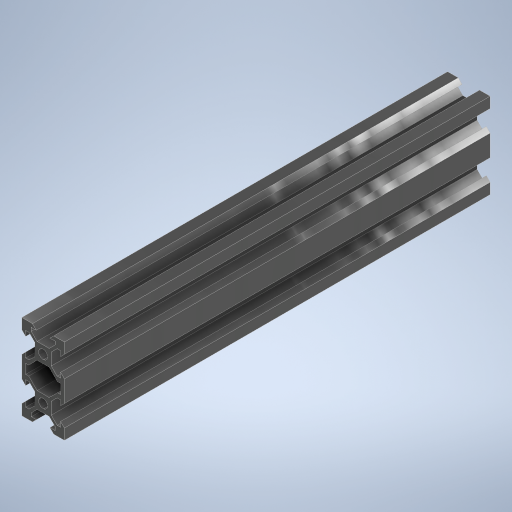
# Autodesk Inventor part: AP20x20
Saved by Autodesk Inventor 2024.2 (Build 282272000, 272)
## iProperties
Created: 2024-08-13
Part Number: AP20x20
Material: Generic
Document SubType Name: Modeling
Designer: Admin
Density: 1 g/cm^3
Appearance: Dark Gray
Author: Admin
Autodesk Inventor part; units mm, degrees
ref_plane "YZ Plane" through (0, 0, 0) normal (1, 0, 0) x (0, 1, 0)
ref_plane "XZ Plane" through (0, 0, 0) normal (0, 1, 0) x (-1, 0, 0)
ref_plane "XY Plane" through (0, 0, 0) normal (0, 0, 1) x (1, 0, 0)
sketch "Sketch1" plane through (0, 0, 0) normal (0, 0, 1) x (1, 0, 0)
  line L0 (-10, -10) -> (-5.6, -10)
  line L1 (-10, -5.6) -> (-10, -10)
  line L2 (-5.6, -10) -> (-5, -10)
  line L3 (-3.2, -8.2) -> (-5.6, -8.2)
  line L4 (-2.8351, -3.825) -> (-5.6, -6.5899)
  line L5 (-3.825, -2.8351) -> (-6.5899, -5.6)
  line L6 (0, 0) -> (0, -11) construction
  line L7 (0, 0) -> (-12, 0) construction
  line L8 (-3.2, -8.2) -> (-5, -10)
  line L9 (-6.5899, -5.6) -> (-8.2, -5.6)
  line L10 (-10, -5.6) -> (-10, -5)
  line L11 (-10, -5) -> (-8.2, -3.2)
  line L12 (-8.2, -3.2) -> (-8.2, -5.6)
  line L13 (-5.6, -8.2) -> (-5.6, -6.5899)
  arc A0 (-2.15, 0) -> (0, -2.15) centre (0, 0) ccw
  line L14 (0, 0) -> (-3.825, 0)
  line L15 (-3.825, 0) -> (-3.825, -2.8351)
  line L16 (-2.8351, -3.825) -> (0, -3.825)
  line L17 (0, -3.825) -> (0, 0)
  line L18 (-2.8351, -3.825) -> (-3.825, -3.825) construction
  line L19 (-3.825, -3.825) -> (-3.825, -2.8351) construction
  line L20 (3.825, -2.8351) -> (3.825, -3.825) construction
  line L21 (3.825, -2.8351) -> (3.825, 0)
  line L22 (3.825, -3.825) -> (2.8351, -3.825) construction
  line L23 (3.825, 0) -> (0, 0)
  line L24 (0, -3.825) -> (2.8351, -3.825)
  arc A1 (0, -2.15) -> (2.15, 0) centre (0, 0) ccw
  line L25 (0, 0) -> (0, -3.825)
  line L26 (2.8351, -3.825) -> (5.6, -6.5899)
  line L27 (0, 0) -> (0, -12) construction
  line L28 (0, 0) -> (11, 0) construction
  line L29 (3.825, -2.8351) -> (6.5899, -5.6)
  line L30 (8.2, -3.2) -> (8.2, -5.6)
  line L31 (10, -5.6) -> (10, -5)
  line L32 (8.2, -3.2) -> (10, -5)
  line L33 (8.2, -5.6) -> (6.5899, -5.6)
  line L34 (5.6, -6.5899) -> (5.6, -8.2)
  line L35 (10, -10) -> (10, -5.6)
  line L36 (5.6, -10) -> (10, -10)
  line L37 (3.2, -8.2) -> (5.6, -8.2)
  line L38 (5, -10) -> (3.2, -8.2)
  line L39 (5.6, -10) -> (5, -10)
  line L40 (2.8351, 3.825) -> (3.825, 3.825) construction
  line L41 (2.8351, 3.825) -> (0, 3.825)
  line L42 (3.825, 3.825) -> (3.825, 2.8351) construction
  line L43 (0, 3.825) -> (0, 0)
  line L44 (3.825, 0) -> (3.825, 2.8351)
  arc A2 (2.15, 0) -> (0, 2.15) centre (0, 0) ccw
  line L45 (0, 0) -> (3.825, 0)
  line L46 (3.825, 2.8351) -> (6.5899, 5.6)
  line L47 (0, 0) -> (12, 0) construction
  line L48 (0, 0) -> (0, 11) construction
  line L49 (2.8351, 3.825) -> (5.6, 6.5899)
  line L50 (3.2, 8.2) -> (5.6, 8.2)
  line L51 (5.6, 10) -> (5, 10)
  line L52 (3.2, 8.2) -> (5, 10)
  line L53 (5.6, 8.2) -> (5.6, 6.5899)
  line L54 (6.5899, 5.6) -> (8.2, 5.6)
  line L55 (10, 10) -> (5.6, 10)
  line L56 (10, 5.6) -> (10, 10)
  line L57 (8.2, 3.2) -> (8.2, 5.6)
  line L58 (10, 5) -> (8.2, 3.2)
  line L59 (10, 5.6) -> (10, 5)
  line L60 (-3.825, 2.8351) -> (-3.825, 3.825) construction
  line L61 (-3.825, 2.8351) -> (-3.825, 0)
  line L62 (-3.825, 3.825) -> (-2.8351, 3.825) construction
  line L63 (-3.825, 0) -> (0, 0)
  line L64 (0, 3.825) -> (-2.8351, 3.825)
  arc A3 (0, 2.15) -> (-2.15, 0) centre (0, 0) ccw
  line L65 (0, 0) -> (0, 3.825)
  line L66 (-2.8351, 3.825) -> (-5.6, 6.5899)
  line L67 (0, 0) -> (0, 12) construction
  line L68 (0, 0) -> (-11, 0) construction
  line L69 (-3.825, 2.8351) -> (-6.5899, 5.6)
  line L70 (-8.2, 3.2) -> (-8.2, 5.6)
  line L71 (-10, 5.6) -> (-10, 5)
  line L72 (-8.2, 3.2) -> (-10, 5)
  line L73 (-8.2, 5.6) -> (-6.5899, 5.6)
  line L74 (-5.6, 6.5899) -> (-5.6, 8.2)
  line L75 (-10, 10) -> (-10, 5.6)
  line L76 (-5.6, 10) -> (-10, 10)
  line L77 (-3.2, 8.2) -> (-5.6, 8.2)
  line L78 (-5, 10) -> (-3.2, 8.2)
  line L79 (-5.6, 10) -> (-5, 10)
  point P0 (0, 2.15)
  point P1 (2.15, 0)
  point P2 (0, -2.15)
  dimension "d16" = 10
  dimension "d19" = 3.2
  dimension "d21" = 4.4
  dimension "d22" = 4.4
  dimension "d24" = 45
  dimension "d25" = 1.8
  dimension "d27" = 1.8
  dimension "d28" = 45
  dimension "d29" = 3.2
  dimension "d31" = 1.4
  dimension "d33" = 2.15
  dimension "d34" = 3.825
  dimension "d35" = 3.825
  dimension "d36" = 135
  dimension "d39" = 360
  constraints: 160 end point, 10 coincident, 8 point on circle, 8 point on line, 6 horizontal, 4 centre point, 3 parallel, 3 vertical, 2 perpendicular, 179 other
  measures "d16" distance between parallel lines of L6 L1
  measures "d19" distance from line of L6 L3.start
  measures "d21" distance of L0.start L0.end
  measures "d22" distance of L1.start L0.start
  measures "d24" angle of L8 L3
  measures "d25" distance between parallel lines of L2 L3
  measures "d27" distance between parallel lines of L10 L12
  measures "d28" angle of L12 L11
  measures "d29" distance from line of L11.end L7
  measures "d31" distance between parallel lines of L5 L4
  measures "d33" radius of A0
  measures "d34" distance of L16.end L18.end
  measures "d35" distance of L18.end L14.end
  measures "d36" angle of L16 L4
extrude "Extrusion1" add sketch "Sketch1" along normal blind 200 contours L1 L10 L11 L12 L9 L5 L15 L14 A0 L17 L16 L4 L13 L3 L8 L2 L0 | L17 A1 L23 L21 L29 L33 L30 L32 L31 L35 L36 L39 L38 L37 L34 L26 L24 | L61 L69 L73 L70 L72 L71 L75 L76 L79 L78 L77 L74 L66 L64 L43 A3 L14 | A2 L43 L41 L49 L53 L50 L52 L51 L55 L56 L59 L58 L57 L54 L46 L44 L23
pattern_linear "Rectangular Pattern1" count 2 spacing 20 along (0, -1, 0) of "Extrusion1"
sketch "Sketch2" plane through (0, 0, 200) normal (0, 0, 1) x (1, 0, 0)
  line L0 (3.2, -8.2) -> (5, -10) projected
  line L1 (-3.2, -11.8) -> (-5, -10) projected
  line L2 (5, -10) -> (-5, -10) construction
  line L3 (-8.2, -12.25) -> (8.2, -12.25)
  line L4 (8.2, -12.25) -> (8.2, -7.75)
  line L5 (8.2, -7.75) -> (-8.2, -7.75)
  line L6 (-8.2, -7.75) -> (-8.2, -12.25)
  line L7 (-8.2, -12.25) -> (8.2, -7.75) construction
  line L8 (8.2, -12.25) -> (-8.2, -7.75) construction
  line L9 (10, -15) -> (10, -5) projected
  line L10 (5.6, -6.5899) -> (5.6, -8.2) projected
  line L11 (5.6, -6.5899) -> (6.7601, -7.75)
  line L12 (-5.6, -6.5899) -> (-2.8351, -3.825) projected
  line L13 (-5.6, -6.5899) -> (-6.7601, -7.75)
  line L14 (5.6, -13.4101) -> (6.7601, -12.25)
  line L15 (-5.6, -13.4101) -> (-6.7601, -12.25)
  line L16 (-5.6, -6.5899) -> (-5.6, -7.75)
  line L17 (-5.6, -8.2) -> (-5.6, -6.5899) projected
  line L18 (5.6, -6.5899) -> (5.6, -7.75)
  line L19 (-5.6, -11.8) -> (-5.6, -13.4101)
  line L20 (5.6, -13.4101) -> (5.6, -12.25)
  point P0 (0, 0)
  point P1 (0, -10)
  point P2 (-5.6, -12.25)
  dimension "d46" = 4.5
  dimension "d50" = 1.8
  constraints: 30 end point, 6 point on line, 6 symmetric about line, 3 midpoint, 2 horizontal, 2 parallel, 1 collinear, 1 perpendicular
  measures "d46" distance of L3.end L4.end
  measures "d50" distance between parallel lines of L4 L9
extrude "Extrusion2" cut sketch "Sketch2" against normal through all
body "Solid1"
